Autodesk Inventor part; units mm, degrees
(part 2 of 2)
sketch "Sketch14" plane through (-31.074, -17.5601, 10.9) normal (0, -1, 0) x (1, 0, 0)
  line L0 (11.262, -18.5) -> (6.69, -18.5) projected
  line L1 (6.69, -18.5) -> (4, -18.5) projected
  line L2 (4, -18.5) -> (0, -18.5) projected
  line L3 (0, -18.5) -> (6.79, -18.5) projected
  line L4 (6.79, -18.5) -> (11.152, -18.5) projected
  line L5 (11.152, -18.5) -> (12.152, -18.5) projected
  line L6 (12.152, -18.5) -> (13.652, -18.5) projected
  line L7 (13.652, -18.5) -> (11.262, -18.5) projected
  line L8 (0, -18.5) -> (0, 0) projected
  line L9 (0, 1) -> (0, -18.5) projected
  line L10 (4, -10.9) -> (5.5, -10.9) projected
  line L11 (5.5, -10.9) -> (4, -10.9) projected
  line L12 (5.301, -10.9) -> (5.5, -10.9) projected
  line L13 (5.5, -10.9) -> (5.301, -10.9) projected
  line L14 (4, -18.5) -> (0, -18.5)
  line L15 (0, -18.5) -> (0, -10.9)
  line L16 (0, -10.9) -> (4, -10.9)
  line L17 (3.15, -10.9) -> (3.15, -18.5)
  line L18 (0, -18.5) -> (6.79, -18.5) projected
  line L19 (0, 0) -> (0, -18.5) projected
  line L20 (0, 1) -> (0, -18.5) projected
  line L21 (4, -18.5) -> (0, -18.5) projected
  line L22 (0, -18.5) -> (4, -18.5) projected
  point P0 (31.074, -10.9)
  point P1 (0, -10.9)
  point P2 (4.15, -12.9)
  dimension "d108" = 1
  constraints: 8 end point, 2 perpendicular, 2 point on line, 1 collinear, 1 horizontal, 1 parallel, 3 other
  measures "d108" distance from line of L17 point (4.15, -12.9)
extrude "Extrusion14" add sketch "Sketch14" along normal up to surface (10 mm away)
sketch "Sketch9" plane through (0, 0, 11.9) normal (0, 0, 1) x (1, 0, 0)
  circle A0 centre (17.787, -22.5201) radius 3.75 projected
  circle A1 centre (17.787, -22.5201) radius 11.05
  point P0 (0, 0)
  dimension "d76" = 22.1
  constraints: 1 centre point, 1 coincident
  measures "d76" diameter of A1
extrude "encoder knob hole" cut sketch "Sketch9" against normal blind 4
sketch "Sketch10" plane through (19.812, 17.7459, -7.6) normal (0, -1, 0) x (1, 0, 0)
  line L0 (7.262, 6) -> (7.262, 0) projected
  line L1 (7.262, 0) -> (4.572, 0) projected
  line L2 (4.572, 6) -> (7.262, 6) projected
  line L3 (-46.886, 6) -> (-44.196, 6) projected
  line L4 (-44.196, 0) -> (-46.886, 0) projected
  line L5 (7.262, 1.5) -> (8.762, 3.4199)
  line L6 (8.762, 3.4199) -> (7.262, 5.3398)
  line L7 (-46.736, 1.5) -> (-48.236, 3.4199)
  line L8 (-48.236, 3.4199) -> (-46.736, 5.3398)
  line L9 (-46.736, 1.5) -> (-46.736, 5.3398)
  line L10 (-46.736, 6) -> (-46.736, 7.6) projected
  point P0 (-19.812, 7.6)
  point P1 (-46.8353, 0)
  dimension "d83" = 1.5
  dimension "d93" = 38
  dimension "d94" = 38
  dimension "d96" = 1.5
  dimension "d109" = 38
  dimension "d110" = 38
  dimension "d111" = 1.5
  dimension "d112" = 1.5
  constraints: 10 end point, 2 point on line, 1 collinear
  measures "d83" distance of L0.end L5.start
  measures "d93" angle of L0 L5
  measures "d94" angle of L0 L6
  measures "d96" distance from line of L0 L5.end
  measures "d109" angle of L8 L9
  measures "d110" angle of L7 L9
  measures "d111" distance from line of L9 L7.end
  measures "d112" distance from line of L4 L7.start
extrude "Extrusion11" cut sketch "Sketch10" along normal through all
sketch "Sketch11" plane through (0, 0, -1.6) normal (0, 0, -1) x (-1, 0, 0)
  line L0 (17.074, -31.6301) -> (-17.074, -31.6301)
  line L1 (-17.074, -31.6301) -> (-17.074, -33.0301)
  line L2 (-17.074, -33.0301) -> (17.074, -33.0301)
  line L3 (17.074, -33.0301) -> (17.074, -31.6301)
  line L4 (-27.074, -33.7654) -> (-27.074, 16.5559) projected
  line L5 (-24.384, -34.3301) -> (24.384, -34.3301) projected
  line L6 (24.384, -30.3301) -> (-24.384, -30.3301) projected
  line L7 (27.074, -27.5601) -> (27.074, -33.7654) projected
  point P0 (0, 0)
  point P1 (27.074, -28.1601)
  dimension "d97" = 10
  dimension "d99" = 1.3
  dimension "d100" = 1.3
  dimension "d124" = 10
  constraints: 8 end point, 2 parallel, 1 horizontal, 1 perpendicular
  measures "d97" distance between parallel lines of L4 L1
  measures "d99" distance between parallel lines of L5 L2
  measures "d100" distance between parallel lines of L6 L0
  measures "d124" distance between parallel lines of L7 L3
extrude "Extrusion12" cut sketch "Sketch11" against normal blind 2
chamfer "Chamfer2" distance 0.5 angle 45 2 edges at (0, -33.0301, -1.6) (0, -31.6301, -1.6)
sketch "Sketch15" plane through (-14.732, 33.4699, -7.6) normal (0, -1, 0) x (1, 0, 0)
  line L0 (3, 1.4) -> (26.464, 1.4)
  line L1 (26.464, 1.4) -> (26.464, 2.6)
  line L2 (26.464, 2.6) -> (3, 2.6)
  line L3 (3, 2.6) -> (3, 1.4)
  line L4 (29.464, 13.5) -> (29.464, 0) projected
  line L5 (0, 13.5) -> (0, 0) projected
  line L6 (29.464, 0) -> (0, 0) projected
  point P0 (14.732, 7.6)
  dimension "d117" = 3
  dimension "d118" = 3
  dimension "d125" = 1.4
  dimension "d126" = 1.2
  constraints: 8 end point, 2 parallel, 1 horizontal, 1 perpendicular
  measures "d117" distance between parallel lines of L4 L1
  measures "d118" distance between parallel lines of L5 L3
  measures "d125" distance between parallel lines of L6 L0
  measures "d126" distance between parallel lines of L2 L0
extrude "Extrusion15" cut sketch "Sketch15" against normal blind 2
sketch "Sketch16" plane through (0, 0, 0) normal (0, 0, 1) x (1, 0, 0)
  line L0 (10.422, 31.4699) -> (2.422, 31.4699)
  line L1 (2.422, 31.4699) -> (2.422, 13.4699)
  line L2 (2.422, 13.4699) -> (10.422, 13.4699)
  line L3 (10.422, 13.4699) -> (10.422, 31.4699)
  line L4 (17.422, 21.6359) -> (17.422, 22.2079) projected
  line L5 (14.732, 33.4699) -> (-14.732, 33.4699) projected
  point P0 (0, 0)
  dimension "d127" = 7
  dimension "d128" = 8
  dimension "d129" = 2
  dimension "d130" = 18
  constraints: 8 end point, 2 parallel, 1 horizontal, 1 perpendicular
  measures "d127" distance between parallel lines of L4 L3
  measures "d128" distance between parallel lines of L3 L1
  measures "d129" distance between parallel lines of L5 L0
  measures "d130" distance between parallel lines of L0 L2
extrude "Extrusion16" cut sketch "Sketch16" along normal blind 8
sketch "Sketch17" plane through (0, 0, 11.9) normal (0, 0, 1) x (1, 0, 0)
  line L0 (-17.8742, 27.8081) -> (4.7876, 27.8081) construction
  line L1 (4.7876, 27.8081) -> (4.7876, 16.8039) construction
  line L2 (4.7876, 16.8039) -> (-17.8742, 16.8039) construction
  line L3 (-17.8742, 16.8039) -> (-17.8742, 27.8081) construction
  line L4 (9.2661, 27.8081) -> (25.0585, 27.8081) construction
  line L5 (25.0585, 27.8081) -> (25.0585, 16.6819) construction
  line L6 (25.0585, 16.6819) -> (9.2661, 16.6819) construction
  line L7 (9.2661, 16.6819) -> (9.2661, 27.8081) construction
  line L8 (-27.8134, 1.6674) -> (-10.9826, 1.6674) construction
  line L9 (-10.9826, 1.6674) -> (-10.9826, -10.8764) construction
  line L10 (-10.9826, -10.8764) -> (-27.8134, -10.8764) construction
  line L11 (-27.8134, -10.8764) -> (-27.8134, 1.6674) construction
  line L12 (-27.8134, -28.2577) -> (-16.1423, -28.2577) construction
  line L13 (-16.1423, -28.2577) -> (-16.1423, -31.3671) construction
  line L14 (-16.1423, -31.3671) -> (-27.8134, -31.3671) construction
  line L15 (-27.8134, -31.3671) -> (-27.8134, -28.2577) construction
  line L16 (-16.0403, 24.7581) -> (-17.6814, 24.7581)
  line L17 (-17.6814, 24.7581) -> (-17.6814, 25.2895)
  line L18 (-17.6814, 25.2895) -> (-17.244, 25.2895)
  line L19 (-17.244, 25.2895) -> (-17.244, 27.2767)
  line L20 (-17.244, 27.2767) -> (-17.6814, 27.2767)
  line L21 (-17.6814, 27.2767) -> (-17.6814, 27.8081)
  line L22 (-17.6814, 27.8081) -> (-16.0403, 27.8081)
  line L23 (-16.0403, 27.8081) -> (-16.0403, 27.2767)
  line L24 (-16.0403, 27.2767) -> (-16.4778, 27.2767)
  line L25 (-16.4778, 27.2767) -> (-16.4778, 25.2895)
  line L26 (-16.4778, 25.2895) -> (-16.0403, 25.2895)
  line L27 (-16.0403, 25.2895) -> (-16.0403, 24.7581)
  line L28 (-12.9186, 24.7581) -> (-13.6551, 24.7581)
  line L29 (-13.6551, 24.7581) -> (-14.8316, 26.8837)
  line L30 (-14.8316, 26.8837) -> (-14.8316, 24.7581)
  line L31 (-14.8316, 24.7581) -> (-15.5311, 24.7581)
  line L32 (-15.5311, 24.7581) -> (-15.5311, 27.8081)
  line L33 (-15.5311, 27.8081) -> (-14.5919, 27.8081)
  line L34 (-14.5919, 27.8081) -> (-13.6181, 26.0606)
  line L35 (-13.6181, 26.0606) -> (-13.6181, 27.8081)
  line L36 (-13.6181, 27.8081) -> (-12.9186, 27.8081)
  line L37 (-12.9186, 27.8081) -> (-12.9186, 24.7581)
  line L38 (-14.8391, 20.8165) -> (-15.887, 20.8165)
  line L39 (-15.887, 20.8165) -> (-15.887, 19.7759)
  line L40 (-15.887, 19.7759) -> (-16.4283, 19.7759)
  line L41 (-16.4283, 19.7759) -> (-16.4283, 20.8165)
  line L42 (-16.4283, 20.8165) -> (-17.4763, 20.8165)
  line L43 (-17.4763, 20.8165) -> (-17.4763, 21.3454)
  line L44 (-17.4763, 21.3454) -> (-16.4283, 21.3454)
  line L45 (-16.4283, 21.3454) -> (-16.4283, 22.3859)
  line L46 (-16.4283, 22.3859) -> (-15.887, 22.3859)
  line L47 (-15.887, 22.3859) -> (-15.887, 21.3454)
  line L48 (-15.887, 21.3454) -> (-14.8391, 21.3454)
  line L49 (-14.8391, 21.3454) -> (-14.8391, 20.8165)
  line L50 (-12.0263, 19.7363) -> (-14.0407, 19.7363)
  line L51 (-14.0407, 19.7363) -> (-14.0407, 20.2677)
  line L52 (-14.0407, 20.2677) -> (-13.3981, 20.2677)
  line L53 (-13.3981, 20.2677) -> (-13.3981, 21.8817)
  line L54 (-13.3981, 21.8817) -> (-14.0407, 21.8817)
  line L55 (-14.0407, 21.8817) -> (-14.0407, 22.3785)
  spline S0 degree 2 poles (-14.0407, 22.3785) (-13.8998, 22.3785) (-13.6205, 22.4156) (-13.5365, 22.4551) knots 0 0 0 1 2 2 2
  spline S1 degree 2 poles (-13.5365, 22.4551) (-13.4401, 22.5046) (-13.3314, 22.6702) (-13.3215, 22.7938) knots 0 0 0 1 2 2 2
  line L56 (-13.3215, 22.7938) -> (-12.6541, 22.7938)
  line L57 (-12.6541, 22.7938) -> (-12.6541, 20.2677)
  line L58 (-12.6541, 20.2677) -> (-12.0263, 20.2677)
  line L59 (-12.0263, 20.2677) -> (-12.0263, 19.7363)
  line L60 (-9.3545, 19.7363) -> (-11.3689, 19.7363)
  line L61 (-11.3689, 19.7363) -> (-11.3689, 20.2677)
  line L62 (-11.3689, 20.2677) -> (-10.7263, 20.2677)
  line L63 (-10.7263, 20.2677) -> (-10.7263, 21.8817)
  line L64 (-10.7263, 21.8817) -> (-11.3689, 21.8817)
  line L65 (-11.3689, 21.8817) -> (-11.3689, 22.3785)
  spline S2 degree 2 poles (-11.3689, 22.3785) (-11.228, 22.3785) (-10.9487, 22.4156) (-10.8647, 22.4551) knots 0 0 0 1 2 2 2
  spline S3 degree 2 poles (-10.8647, 22.4551) (-10.7683, 22.5046) (-10.6595, 22.6702) (-10.6496, 22.7938) knots 0 0 0 1 2 2 2
  line L66 (-10.6496, 22.7938) -> (-9.9823, 22.7938)
  line L67 (-9.9823, 22.7938) -> (-9.9823, 20.2677)
  line L68 (-9.9823, 20.2677) -> (-9.3545, 20.2677)
  line L69 (-9.3545, 20.2677) -> (-9.3545, 19.7363)
  line L70 (-6.7321, 19.7363) -> (-7.4489, 19.7363)
  line L71 (-7.4489, 19.7363) -> (-7.4489, 19.9761)
  spline S4 degree 2 poles (-7.4489, 19.9761) (-7.5181, 19.9192) (-7.696, 19.7882) (-7.7652, 19.7536) knots 0 0 0 1 2 2 2
  spline S5 degree 2 poles (-7.7652, 19.7536) (-7.8493, 19.7141) (-8.0173, 19.6721) (-8.1335, 19.6721) knots 0 0 0 1 2 2 2
  spline S6 degree 2 poles (-8.1335, 19.6721) (-8.5265, 19.6721) (-8.9862, 20.3246) (-8.9862, 20.8684) knots 0 0 0 1 2 2 2
  spline S7 degree 2 poles (-8.9862, 20.8684) (-8.9862, 21.1699) (-8.8305, 21.6123) (-8.6946, 21.7754) knots 0 0 0 1 2 2 2
  spline S8 degree 2 poles (-8.6946, 21.7754) (-8.5685, 21.9262) (-8.2126, 22.0992) (-8.0149, 22.0992) knots 0 0 0 1 2 2 2
  spline S9 degree 2 poles (-8.0149, 22.0992) (-7.8344, 22.0992) (-7.6021, 22.0226) (-7.4489, 21.9435) knots 0 0 0 1 2 2 2
  line L72 (-7.4489, 21.9435) -> (-7.4489, 22.9223)
  line L73 (-7.4489, 22.9223) -> (-6.7321, 22.9223)
  line L74 (-6.7321, 22.9223) -> (-6.7321, 19.7363)
  line L75 (-7.4489, 20.3691) -> (-7.4489, 21.4986)
  spline S10 degree 2 poles (-7.4489, 21.4986) (-7.5008, 21.5258) (-7.6738, 21.5604) (-7.7356, 21.5604) knots 0 0 0 1 2 2 2
  spline S11 degree 2 poles (-7.7356, 21.5604) (-7.9926, 21.5604) (-8.2521, 21.1996) (-8.2521, 20.8758) knots 0 0 0 1 2 2 2
  spline S12 degree 2 poles (-8.2521, 20.8758) (-8.2521, 20.5347) (-8.0445, 20.2307) (-7.8147, 20.2307) knots 0 0 0 1 2 2 2
  spline S13 degree 2 poles (-7.8147, 20.2307) (-7.7207, 20.2307) (-7.528, 20.3048) (-7.4489, 20.3691) knots 0 0 0 1 2 2 2
  spline S14 degree 2 poles (-3.7043, 20.6706) (-3.7043, 20.4432) (-3.8774, 20.0997) (-4.0207, 19.986) knots 0 0 0 1 2 2 2
  spline S15 degree 2 poles (-4.0207, 19.986) (-4.1937, 19.85) (-4.604, 19.7363) (-4.9229, 19.7363) knots 0 0 0 1 2 2 2
  line L76 (-4.9229, 19.7363) -> (-6.1414, 19.7363)
  line L77 (-6.1414, 19.7363) -> (-6.1414, 22.7863)
  line L78 (-6.1414, 22.7863) -> (-5.0662, 22.7863)
  spline S16 degree 2 poles (-5.0662, 22.7863) (-4.7301, 22.7863) (-4.384, 22.7344) (-4.2333, 22.6529) knots 0 0 0 1 2 2 2
  spline S17 degree 2 poles (-4.2333, 22.6529) (-4.0677, 22.5664) (-3.907, 22.2698) (-3.907, 22.077) knots 0 0 0 1 2 2 2
  spline S18 degree 2 poles (-3.907, 22.077) (-3.907, 21.8545) (-4.1295, 21.506) (-4.3272, 21.4245) knots 0 0 0 1 2 2 2
  line L79 (-4.3272, 21.4245) -> (-4.3272, 21.4096)
  spline S19 degree 2 poles (-4.3272, 21.4096) (-4.043, 21.3503) (-3.7043, 20.9821) (-3.7043, 20.6706) knots 0 0 0 1 2 2 2
  spline S20 degree 2 poles (-4.4953, 20.683) (-4.4953, 20.8263) (-4.609, 20.987) (-4.7227, 21.029) knots 0 0 0 1 2 2 2
  spline S21 degree 2 poles (-4.7227, 21.029) (-4.7919, 21.0562) (-5.0365, 21.0611) (-5.2392, 21.0611) knots 0 0 0 1 2 2 2
  line L80 (-5.2392, 21.0611) -> (-5.3801, 21.0611)
  line L81 (-5.3801, 21.0611) -> (-5.3801, 20.2925)
  line L82 (-5.3801, 20.2925) -> (-5.3381, 20.2925)
  spline S22 degree 2 poles (-5.3381, 20.2925) (-5.0415, 20.2925) (-4.8141, 20.2999) (-4.6955, 20.3518) knots 0 0 0 1 2 2 2
  spline S23 degree 2 poles (-4.6955, 20.3518) (-4.5917, 20.3987) (-4.4953, 20.5718) (-4.4953, 20.683) knots 0 0 0 1 2 2 2
  spline S24 degree 2 poles (-4.6856, 21.9262) (-4.6856, 22.0004) (-4.7622, 22.1561) (-4.8413, 22.1907) knots 0 0 0 1 2 2 2
  spline S25 degree 2 poles (-4.8413, 22.1907) (-4.9154, 22.2253) (-5.1231, 22.2302) (-5.3282, 22.2302) knots 0 0 0 1 2 2 2
  line L83 (-5.3282, 22.2302) -> (-5.3801, 22.2302)
  line L84 (-5.3801, 22.2302) -> (-5.3801, 21.5827)
  line L85 (-5.3801, 21.5827) -> (-5.2837, 21.5827)
  spline S26 degree 2 poles (-5.2837, 21.5827) (-5.0885, 21.5827) (-4.9303, 21.5901) (-4.8462, 21.6296) knots 0 0 0 1 2 2 2
  spline S27 degree 2 poles (-4.8462, 21.6296) (-4.7548, 21.6741) (-4.6856, 21.8249) (-4.6856, 21.9262) knots 0 0 0 1 2 2 2
  line L86 (-0.5604, 19.7363) -> (-0.5604, 20.8857)
  spline S28 degree 2 poles (-0.5604, 20.8857) (-0.5604, 21.0562) (-0.5728, 21.2885) (-0.6024, 21.3627) knots 0 0 0 1 2 2 2
  spline S29 degree 2 poles (-0.6024, 21.3627) (-0.6346, 21.4368) (-0.7631, 21.5036) (-0.8793, 21.5036) knots 0 0 0 1 2 2 2
  spline S30 degree 2 poles (-0.8793, 21.5036) (-0.9608, 21.5036) (-1.119, 21.4319) (-1.2129, 21.3652) knots 0 0 0 1 2 2 2
  line L87 (-1.2129, 21.3652) -> (-1.2129, 19.7363)
  line L88 (-1.2129, 19.7363) -> (-1.9346, 19.7363)
  line L89 (-1.9346, 19.7363) -> (-1.9346, 20.8857)
  spline S31 degree 2 poles (-1.9346, 20.8857) (-1.9346, 21.0537) (-1.9495, 21.2885) (-1.9791, 21.3627) knots 0 0 0 1 2 2 2
  spline S32 degree 2 poles (-1.9791, 21.3627) (-2.0113, 21.4368) (-2.1398, 21.5036) (-2.256, 21.5036) knots 0 0 0 1 2 2 2
  spline S33 degree 2 poles (-2.256, 21.5036) (-2.3425, 21.5036) (-2.513, 21.422) (-2.5921, 21.3652) knots 0 0 0 1 2 2 2
  line L90 (-2.5921, 21.3652) -> (-2.5921, 19.7363)
  line L91 (-2.5921, 19.7363) -> (-3.3089, 19.7363)
  line L92 (-3.3089, 19.7363) -> (-3.3089, 22.0374)
  line L93 (-3.3089, 22.0374) -> (-2.5921, 22.0374)
  line L94 (-2.5921, 22.0374) -> (-2.5921, 21.7829)
  spline S34 degree 2 poles (-2.5921, 21.7829) (-2.4166, 21.9312) (-2.1027, 22.0992) (-1.9075, 22.0992) knots 0 0 0 1 2 2 2
  spline S35 degree 2 poles (-1.9075, 22.0992) (-1.6974, 22.0992) (-1.3761, 21.899) (-1.292, 21.6988) knots 0 0 0 1 2 2 2
  spline S36 degree 2 poles (-1.292, 21.6988) (-1.0869, 21.8916) (-0.7211, 22.0992) (-0.5332, 22.0992) knots 0 0 0 1 2 2 2
  spline S37 degree 2 poles (-0.5332, 22.0992) (-0.3726, 22.0992) (-0.118, 21.9979) (-0.0315, 21.8941) knots 0 0 0 1 2 2 2
  spline S38 degree 2 poles (-0.0315, 21.8941) (0.0649, 21.7829) (0.1613, 21.4788) (0.1613, 21.2342) knots 0 0 0 1 2 2 2
  line L95 (0.1613, 21.2342) -> (0.1613, 19.7363)
  line L96 (0.1613, 19.7363) -> (-0.5604, 19.7363)
  line L97 (-14.4436, 14.7146) -> (-15.2049, 14.7146)
  line L98 (-15.2049, 14.7146) -> (-15.2049, 16.7364)
  line L99 (-15.2049, 16.7364) -> (-15.7585, 15.4314)
  line L100 (-15.7585, 15.4314) -> (-16.2825, 15.4314)
  line L101 (-16.2825, 15.4314) -> (-16.8361, 16.7364)
  line L102 (-16.8361, 16.7364) -> (-16.8361, 14.7146)
  line L103 (-16.8361, 14.7146) -> (-17.5579, 14.7146)
  line L104 (-17.5579, 14.7146) -> (-17.5579, 17.7646)
  line L105 (-17.5579, 17.7646) -> (-16.6755, 17.7646)
  line L106 (-16.6755, 17.7646) -> (-15.9983, 16.2594)
  line L107 (-15.9983, 16.2594) -> (-15.326, 17.7646)
  line L108 (-15.326, 17.7646) -> (-14.4436, 17.7646)
  line L109 (-14.4436, 17.7646) -> (-14.4436, 14.7146)
  line L110 (-14.1396, 14.7146) -> (-13.1089, 17.7646)
  line L111 (-13.1089, 17.7646) -> (-12.2735, 17.7646)
  line L112 (-12.2735, 17.7646) -> (-11.2428, 14.7146)
  line L113 (-11.2428, 14.7146) -> (-12.0313, 14.7146)
  line L114 (-12.0313, 14.7146) -> (-12.2216, 15.3375)
  line L115 (-12.2216, 15.3375) -> (-13.1806, 15.3375)
  line L116 (-13.1806, 15.3375) -> (-13.3734, 14.7146)
  line L117 (-13.3734, 14.7146) -> (-14.1396, 14.7146)
  line L118 (-12.3897, 15.8911) -> (-12.7011, 16.8995)
  line L119 (-12.7011, 16.8995) -> (-13.015, 15.8911)
  line L120 (-13.015, 15.8911) -> (-12.3897, 15.8911)
  line L121 (-8.3584, 14.7146) -> (-9.2433, 14.7146)
  line L122 (-9.2433, 14.7146) -> (-9.8315, 15.686)
  line L123 (-9.8315, 15.686) -> (-10.4321, 14.7146)
  line L124 (-10.4321, 14.7146) -> (-11.2799, 14.7146)
  line L125 (-11.2799, 14.7146) -> (-10.2888, 16.2495)
  line L126 (-10.2888, 16.2495) -> (-11.2404, 17.7646)
  line L127 (-11.2404, 17.7646) -> (-10.3555, 17.7646)
  line L128 (-10.3555, 17.7646) -> (-9.8043, 16.8427)
  line L129 (-9.8043, 16.8427) -> (-9.2383, 17.7646)
  line L130 (-9.2383, 17.7646) -> (-8.3906, 17.7646)
  line L131 (-8.3906, 17.7646) -> (-9.3471, 16.2816)
  line L132 (-9.3471, 16.2816) -> (-8.3584, 14.7146)
  spline S39 degree 2 poles (12.3581, 26.2188) (12.3581, 25.4773) (11.5671, 24.6296) (10.88, 24.6296) knots 0 0 0 1 2 2 2
  spline S40 degree 2 poles (10.88, 24.6296) (10.1904, 24.6296) (9.4045, 25.4872) (9.4045, 26.2188) knots 0 0 0 1 2 2 2
  spline S41 degree 2 poles (9.4045, 26.2188) (9.4045, 26.9529) (10.1904, 27.8081) (10.88, 27.8081) knots 0 0 0 1 2 2 2
  spline S42 degree 2 poles (10.88, 27.8081) (11.5671, 27.8081) (12.3581, 26.9578) (12.3581, 26.2188) knots 0 0 0 1 2 2 2
  spline S43 degree 2 poles (11.5671, 26.2188) (11.5671, 26.4932) (11.4559, 26.8763) (11.3595, 26.9974) knots 0 0 0 1 2 2 2
  spline S44 degree 2 poles (11.3595, 26.9974) (11.2631, 27.1234) (11.016, 27.2322) (10.8825, 27.2322) knots 0 0 0 1 2 2 2
  spline S45 degree 2 poles (10.8825, 27.2322) (10.7416, 27.2322) (10.5118, 27.1309) (10.4055, 27.0023) knots 0 0 0 1 2 2 2
  spline S46 degree 2 poles (10.4055, 27.0023) (10.3116, 26.8837) (10.1954, 26.4907) (10.1954, 26.2188) knots 0 0 0 1 2 2 2
  spline S47 degree 2 poles (10.1954, 26.2188) (10.1954, 25.9371) (10.3066, 25.5663) (10.403, 25.4403) knots 0 0 0 1 2 2 2
  spline S48 degree 2 poles (10.403, 25.4403) (10.4994, 25.3142) (10.749, 25.2055) (10.8825, 25.2055) knots 0 0 0 1 2 2 2
  spline S49 degree 2 poles (10.8825, 25.2055) (11.0184, 25.2055) (11.2706, 25.3216) (11.362, 25.4452) knots 0 0 0 1 2 2 2
  spline S50 degree 2 poles (11.362, 25.4452) (11.4609, 25.5787) (11.5671, 25.9321) (11.5671, 26.2188) knots 0 0 0 1 2 2 2
  spline S51 degree 2 poles (14.0462, 24.6296) (13.4308, 24.6296) (12.7684, 25.2228) (12.7684, 25.7962) knots 0 0 0 1 2 2 2
  line L133 (12.7684, 25.7962) -> (12.7684, 27.7438)
  line L134 (12.7684, 27.7438) -> (13.5346, 27.7438)
  line L135 (13.5346, 27.7438) -> (13.5346, 25.8407)
  spline S52 degree 2 poles (13.5346, 25.8407) (13.5346, 25.5218) (13.7743, 25.2104) (14.0462, 25.2104) knots 0 0 0 1 2 2 2
  spline S53 degree 2 poles (14.0462, 25.2104) (14.3107, 25.2104) (14.5578, 25.5095) (14.5578, 25.8407) knots 0 0 0 1 2 2 2
  line L136 (14.5578, 25.8407) -> (14.5578, 27.7438)
  line L137 (14.5578, 27.7438) -> (15.324, 27.7438)
  line L138 (15.324, 27.7438) -> (15.324, 25.7986)
  spline S54 degree 2 poles (15.324, 25.7986) (15.324, 25.2351) (14.6789, 24.6296) (14.0462, 24.6296) knots 0 0 0 1 2 2 2
  line L139 (16.4981, 24.6938) -> (16.4981, 27.163)
  line L140 (16.4981, 27.163) -> (15.5959, 27.163)
  line L141 (15.5959, 27.163) -> (15.5959, 27.7438)
  line L142 (15.5959, 27.7438) -> (18.1664, 27.7438)
  line L143 (18.1664, 27.7438) -> (18.1664, 27.163)
  line L144 (18.1664, 27.163) -> (17.2643, 27.163)
  line L145 (17.2643, 27.163) -> (17.2643, 24.6938)
  line L146 (17.2643, 24.6938) -> (16.4981, 24.6938)
  spline S55 degree 2 poles (-24.9512, -1.2689) (-25.1514, -1.3504) (-25.7916, -1.5062) (-26.103, -1.5062) knots 0 0 0 1 2 2 2
  spline S56 degree 2 poles (-26.103, -1.5062) (-26.8223, -1.5062) (-27.675, -0.6757) (-27.675, 0.0856) knots 0 0 0 1 2 2 2
  spline S57 degree 2 poles (-27.675, 0.0856) (-27.675, 0.8024) (-26.8223, 1.6674) (-26.0808, 1.6674) knots 0 0 0 1 2 2 2
  spline S58 degree 2 poles (-26.0808, 1.6674) (-25.6977, 1.6674) (-25.2182, 1.5216) (-24.9636, 1.398) knots 0 0 0 1 2 2 2
  line L147 (-24.9636, 1.398) -> (-24.9636, 0.6812)
  line L148 (-24.9636, 0.6812) -> (-25.0328, 0.6812)
  spline S59 degree 2 poles (-25.0328, 0.6812) (-25.0872, 0.7233) (-25.2948, 0.8839) (-25.3937, 0.9383) knots 0 0 0 1 2 2 2
  spline S60 degree 2 poles (-25.3937, 0.9383) (-25.5074, 1.005) (-25.8089, 1.0989) (-25.977, 1.0989) knots 0 0 0 1 2 2 2
  spline S61 degree 2 poles (-25.977, 1.0989) (-26.1722, 1.0989) (-26.496, 0.9754) (-26.6221, 0.8493) knots 0 0 0 1 2 2 2
  spline S62 degree 2 poles (-26.6221, 0.8493) (-26.7432, 0.7257) (-26.8841, 0.3476) (-26.8841, 0.0979) knots 0 0 0 1 2 2 2
  spline S63 degree 2 poles (-26.8841, 0.0979) (-26.8841, -0.4359) (-26.3477, -0.9451) (-25.8855, -0.9451) knots 0 0 0 1 2 2 2
  spline S64 degree 2 poles (-25.8855, -0.9451) (-25.8435, -0.9451) (-25.7347, -0.9402) (-25.6927, -0.9377) knots 0 0 0 1 2 2 2
  line L149 (-25.6927, -0.9377) -> (-25.6927, -0.3371)
  line L150 (-25.6927, -0.3371) -> (-26.2834, -0.3371)
  line L151 (-26.2834, -0.3371) -> (-26.2834, 0.2339)
  line L152 (-26.2834, 0.2339) -> (-24.9512, 0.2339)
  line L153 (-24.9512, 0.2339) -> (-24.9512, -1.2689)
  line L154 (-24.7016, -1.4419) -> (-23.6709, 1.6081)
  line L155 (-23.6709, 1.6081) -> (-22.8355, 1.6081)
  line L156 (-22.8355, 1.6081) -> (-21.8048, -1.4419)
  line L157 (-21.8048, -1.4419) -> (-22.5933, -1.4419)
  line L158 (-22.5933, -1.4419) -> (-22.7836, -0.819)
  line L159 (-22.7836, -0.819) -> (-23.7426, -0.819)
  line L160 (-23.7426, -0.819) -> (-23.9354, -1.4419)
  line L161 (-23.9354, -1.4419) -> (-24.7016, -1.4419)
  line L162 (-22.9517, -0.2654) -> (-23.2631, 0.743)
  line L163 (-23.2631, 0.743) -> (-23.577, -0.2654)
  line L164 (-23.577, -0.2654) -> (-22.9517, -0.2654)
  line L165 (-19.9832, -1.4419) -> (-21.6244, -1.4419)
  line L166 (-21.6244, -1.4419) -> (-21.6244, -0.9105)
  line L167 (-21.6244, -0.9105) -> (-21.1869, -0.9105)
  line L168 (-21.1869, -0.9105) -> (-21.1869, 1.0767)
  line L169 (-21.1869, 1.0767) -> (-21.6244, 1.0767)
  line L170 (-21.6244, 1.0767) -> (-21.6244, 1.6081)
  line L171 (-21.6244, 1.6081) -> (-19.9832, 1.6081)
  line L172 (-19.9832, 1.6081) -> (-19.9832, 1.0767)
  line L173 (-19.9832, 1.0767) -> (-20.4207, 1.0767)
  line L174 (-20.4207, 1.0767) -> (-20.4207, -0.9105)
  line L175 (-20.4207, -0.9105) -> (-19.9832, -0.9105)
  line L176 (-19.9832, -0.9105) -> (-19.9832, -1.4419)
  line L177 (-16.8616, -1.4419) -> (-17.5981, -1.4419)
  line L178 (-17.5981, -1.4419) -> (-18.7746, 0.6837)
  line L179 (-18.7746, 0.6837) -> (-18.7746, -1.4419)
  line L180 (-18.7746, -1.4419) -> (-19.4741, -1.4419)
  line L181 (-19.4741, -1.4419) -> (-19.4741, 1.6081)
  line L182 (-19.4741, 1.6081) -> (-18.5349, 1.6081)
  line L183 (-18.5349, 1.6081) -> (-17.561, -0.1393)
  line L184 (-17.561, -0.1393) -> (-17.561, 1.6081)
  line L185 (-17.561, 1.6081) -> (-16.8616, 1.6081)
  line L186 (-16.8616, 1.6081) -> (-16.8616, -1.4419)
  line L187 (-25.3294, -28.9226) -> (-26.6319, -31.3671)
  line L188 (-26.6319, -31.3671) -> (-27.4822, -31.3671)
  line L189 (-27.4822, -31.3671) -> (-26.1203, -28.893)
  line L190 (-26.1203, -28.893) -> (-27.5736, -28.893)
  line L191 (-27.5736, -28.893) -> (-27.5736, -28.3171)
  line L192 (-27.5736, -28.3171) -> (-25.3294, -28.3171)
  line L193 (-25.3294, -28.3171) -> (-25.3294, -28.9226)
  line L194 (-23.5597, -30.3043) -> (-24.9166, -30.3043)
  line L195 (-24.9166, -30.3043) -> (-24.9166, -29.7358)
  line L196 (-24.9166, -29.7358) -> (-23.5597, -29.7358)
  line L197 (-23.5597, -29.7358) -> (-23.5597, -30.3043)
  line L198 (-20.7816, -31.3671) -> (-23.0234, -31.3671)
  line L199 (-23.0234, -31.3671) -> (-23.0234, -30.8703)
  spline S65 degree 2 poles (-23.0234, -30.8703) (-22.7391, -30.6429) (-22.2843, -30.2425) (-22.1138, -30.062) knots 0 0 0 1 2 2 2
  spline S66 degree 2 poles (-22.1138, -30.062) (-21.8889, -29.8272) (-21.6887, -29.4688) (-21.6887, -29.281) knots 0 0 0 1 2 2 2
  spline S67 degree 2 poles (-21.6887, -29.281) (-21.6887, -29.0684) (-21.9433, -28.841) (-22.1706, -28.841) knots 0 0 0 1 2 2 2
  spline S68 degree 2 poles (-22.1706, -28.841) (-22.2868, -28.841) (-22.4944, -28.8979) (-22.6007, -28.9424) knots 0 0 0 1 2 2 2
  spline S69 degree 2 poles (-22.6007, -28.9424) (-22.7045, -28.9893) (-22.8528, -29.0882) (-22.8899, -29.1129) knots 0 0 0 1 2 2 2
  line L200 (-22.8899, -29.1129) -> (-22.9492, -29.1129)
  line L201 (-22.9492, -29.1129) -> (-22.9492, -28.4481)
  spline S70 degree 2 poles (-22.9492, -28.4481) (-22.8207, -28.3863) (-22.272, -28.2577) (-22.0174, -28.2577) knots 0 0 0 1 2 2 2
  spline S71 degree 2 poles (-22.0174, -28.2577) (-21.4736, -28.2577) (-20.9151, -28.7422) (-20.9151, -29.1797) knots 0 0 0 1 2 2 2
  spline S72 degree 2 poles (-20.9151, -29.1797) (-20.9151, -29.4491) (-21.1696, -29.9681) (-21.4638, -30.2647) knots 0 0 0 1 2 2 2
  spline S73 degree 2 poles (-21.4638, -30.2647) (-21.6491, -30.4476) (-21.9976, -30.7319) (-22.0743, -30.7912) knots 0 0 0 1 2 2 2
  line L202 (-22.0743, -30.7912) -> (-20.7816, -30.7912)
  line L203 (-20.7816, -30.7912) -> (-20.7816, -31.3671)
  spline S74 degree 2 poles (-18.179, -30.3339) (-18.179, -30.5737) (-18.3421, -30.979) (-18.5027, -31.1248) knots 0 0 0 1 2 2 2
  spline S75 degree 2 poles (-18.5027, -31.1248) (-18.6634, -31.2707) (-19.1033, -31.4313) (-19.4247, -31.4313) knots 0 0 0 1 2 2 2
  spline S76 degree 2 poles (-19.4247, -31.4313) (-19.7657, -31.4289) (-20.2551, -31.3176) (-20.4158, -31.246) knots 0 0 0 1 2 2 2
  line L204 (-20.4158, -31.246) -> (-20.4158, -30.5811)
  line L205 (-20.4158, -30.5811) -> (-20.3466, -30.5811)
  spline S77 degree 2 poles (-20.3466, -30.5811) (-20.2873, -30.6132) (-20.1439, -30.6972) (-20.0277, -30.7417) knots 0 0 0 1 2 2 2
  spline S78 degree 2 poles (-20.0277, -30.7417) (-19.919, -30.7838) (-19.6941, -30.8406) (-19.5581, -30.8406) knots 0 0 0 1 2 2 2
  spline S79 degree 2 poles (-19.5581, -30.8406) (-19.4395, -30.8406) (-19.1627, -30.7813) (-19.0786, -30.7022) knots 0 0 0 1 2 2 2
  spline S80 degree 2 poles (-19.0786, -30.7022) (-19.0168, -30.6404) (-18.9476, -30.4896) (-18.9476, -30.3636) knots 0 0 0 1 2 2 2
  spline S81 degree 2 poles (-18.9476, -30.3636) (-18.9476, -30.2548) (-19.0366, -30.1016) (-19.1083, -30.0546) knots 0 0 0 1 2 2 2
  spline S82 degree 2 poles (-19.1083, -30.0546) (-19.2121, -29.9854) (-19.5087, -29.9459) (-19.615, -29.9459) knots 0 0 0 1 2 2 2
  spline S83 degree 2 poles (-19.615, -29.9459) (-19.783, -29.9459) (-20.1019, -30.0002) (-20.2181, -30.0299) knots 0 0 0 1 2 2 2
  line L206 (-20.2181, -30.0299) -> (-20.2848, -30.0299)
  line L207 (-20.2848, -30.0299) -> (-20.2848, -28.3171)
  line L208 (-20.2848, -28.3171) -> (-18.263, -28.3171)
  line L209 (-18.263, -28.3171) -> (-18.263, -28.893)
  line L210 (-18.263, -28.893) -> (-19.5606, -28.893)
  line L211 (-19.5606, -28.893) -> (-19.5606, -29.3996)
  spline S84 degree 2 poles (-19.5606, -29.3996) (-19.4988, -29.3947) (-19.3283, -29.3898) (-19.2813, -29.3898) knots 0 0 0 1 2 2 2
  spline S85 degree 2 poles (-19.2813, -29.3898) (-19.0613, -29.3898) (-18.6906, -29.4787) (-18.5448, -29.5702) knots 0 0 0 1 2 2 2
  spline S86 degree 2 poles (-18.5448, -29.5702) (-18.3717, -29.6839) (-18.179, -30.062) (-18.179, -30.3339) knots 0 0 0 1 2 2 2
  line L212 (-15.1265, -28.3171) -> (-16.1745, -31.3671)
  line L213 (-16.1745, -31.3671) -> (-16.9728, -31.3671)
  line L214 (-16.9728, -31.3671) -> (-18.0208, -28.3171)
  line L215 (-18.0208, -28.3171) -> (-17.2274, -28.3171)
  line L216 (-17.2274, -28.3171) -> (-16.5625, -30.3858)
  line L217 (-16.5625, -30.3858) -> (-15.9001, -28.3171)
  line L218 (-15.9001, -28.3171) -> (-15.1265, -28.3171)
  point P0 (0, 0)
  dimension "d133" = 0
  constraints: 1 collinear, 8 other
  measures "d133" distance between parallel lines of L4 L0
extrude "Extrusion17" cut sketch "Sketch17" against normal blind 1
body "Solid1"
